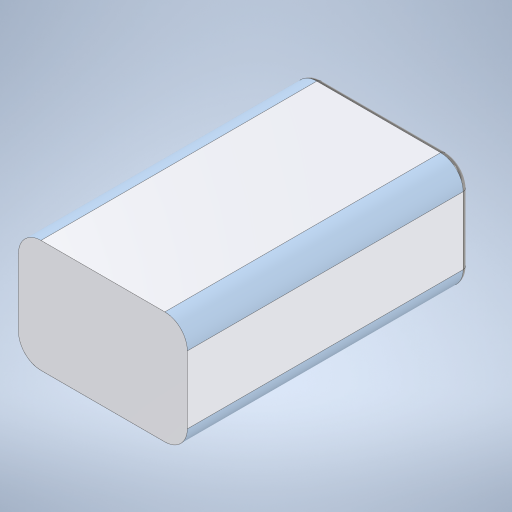
# Autodesk Inventor part: battery eg 26
Saved by Autodesk Inventor 2023 (Build 270158000, 158)
## iProperties
Created: 2023-10-16
Part Number: battery eg 26
Material: Generic
Document SubType Name: Modeling
Designer: user
Density: 1 g/cm^3
Appearance: Default
Author: user
Autodesk Inventor part; units mm, degrees
ref_plane "YZ Plane" through (0, 0, 0) normal (1, 0, 0) x (0, 1, 0)
ref_plane "XZ Plane" through (0, 0, 0) normal (0, 1, 0) x (-1, 0, 0)
ref_plane "XY Plane" through (0, 0, 0) normal (0, 0, 1) x (1, 0, 0)
sketch "Sketch1" plane through (0, 0, 0) normal (0, 0, 1) x (1, 0, 0)
  line L0 (0, 0) -> (150, 0)
  line L1 (150, 0) -> (150, 100)
  line L2 (150, 100) -> (0, 100)
  line L3 (0, 100) -> (0, 0)
  dimension "d0" = 150
  dimension "d1" = 100
  constraints: 8 end point, 2 parallel, 1 horizontal, 1 perpendicular
  measures "d0" distance of L1.end L2.end
  measures "d1" distance of L0.end L1.end
extrude "Extrusion1" add sketch "Sketch1" along normal blind 250
fillet "Fillet1" radius 20 1 edges at (150, 100, 125)
fillet "Fillet2" radius 20 1 edges at (150, 0, 125)
fillet "Fillet3" radius 20 1 edges at (0, 100, 125)
fillet "Fillet4" radius 20 1 edges at (0, 0, 125)
fillet "Fillet5" radius 5 8 edges at (5.8579, 94.1421, 0) (0, 50, 0) (5.8579, 5.8579, 0) (75, 0, 0) (144.1421, 5.8579, 0) (150, 50, 0) (144.1421, 94.1421, 0) (75, 100, 0)
sketch "Sketch2" plane through (20, 0, 250) normal (0, -1, 0) x (1, 0, 0)
  line L0 (110, 0) -> (110, -245) projected
  line L1 (0, -245) -> (0, 0) projected
  line L2 (110, -171.6757) -> (0, -171.6757)
  line L3 (0, -171.6757) -> (0, -166.6757)
  line L4 (0, -166.6757) -> (110, -166.6757)
  line L5 (110, -166.6757) -> (110, -171.6757)
  line L6 (95.3863, -226.2308) -> (70.3863, -226.2308)
  line L7 (70.3863, -226.2308) -> (70.3863, -221.2308)
  line L8 (70.3863, -221.2308) -> (95.3863, -221.2308)
  line L9 (95.3863, -221.2308) -> (95.3863, -226.2308)
  line L10 (37.9599, -226.2308) -> (12.9599, -226.2308)
  line L11 (12.9599, -226.2308) -> (12.9599, -221.2308)
  line L12 (12.9599, -221.2308) -> (37.9599, -221.2308)
  line L13 (37.9599, -221.2308) -> (37.9599, -226.2308)
  line L14 (27.9599, -236.2308) -> (22.9599, -236.2308)
  line L15 (22.9599, -236.2308) -> (22.9599, -211.2308)
  line L16 (22.9599, -211.2308) -> (27.9599, -211.2308)
  line L17 (27.9599, -211.2308) -> (27.9599, -236.2308)
  point P0 (-20, -250)
  point P1 (27.9599, -226.2308)
  point P2 (27.9599, -221.2308)
  point P3 (22.9599, -221.2308)
  point P4 (22.9599, -226.2308)
  dimension "d9" = 25
  dimension "d10" = 5
  dimension "d11" = 5
  dimension "d12" = 25
  dimension "d13" = 10
  dimension "d14" = 10
  dimension "d15" = 5
  dimension "d16" = 25
  dimension "d17" = 5
  constraints: 32 end point, 8 parallel, 4 horizontal, 4 perpendicular, 2 point on line, 1 coincident
  measures "d9" distance of L7.end L8.end
  measures "d10" distance of L6.end L7.end
  measures "d11" distance between parallel lines of L2 L4
  measures "d12" distance of L11.end L12.end
  measures "d13" horizontal distance of L14.start L10.start
  measures "d14" distance from line of L10 L14.start
  measures "d15" distance of L15.end L16.end
  measures "d16" distance of L14.end L15.end
  measures "d17" distance of L10.end L11.end
extrude "Extrusion2" add sketch "Sketch2" along normal blind 5
sketch "Sketch3" plane through (0, 0, 0) normal (0, 0, -1) x (-1, 0, 0)
  line L0 (-20, 100) -> (-130, 100) projected
  line L1 (-150, 80) -> (-150, 20) projected
  circle A0 centre (-110, 50) radius 12.5
  circle A1 centre (-40, 51.4507) radius 12.5
  point P0 (0, 0)
  point P1 (-150, 50)
  dimension "d20" = 50
  dimension "d21" = 40
  dimension "d22" = 70
  dimension "d23" = 25
  dimension "d24" = 25
  constraints: 2 centre point, 2 coincident, 1 midpoint
  measures "d20" distance from line of L0 point (-110, 50)
  measures "d21" distance of point (-150, 50) point (-110, 50)
  measures "d22" horizontal distance of point (-110, 50) point (-40, 51.451)
  measures "d23" diameter of A1
  measures "d24" diameter of A0
extrude "Extrusion3" add sketch "Sketch3" along normal blind 3
sketch "Sketch4" plane through (110, 50, -3) normal (0, 0, -1) x (-1, 0, 0)
  circle A0 centre (0, 0) radius 7.2404
  circle A1 centre (70, 1.4507) radius 12.5 projected
  circle A2 centre (70, 1.4507) radius 7.5
  point P0 (110, -50)
  dimension "d27" = 15
  constraints: 2 centre point, 1 coincident
  measures "d27" diameter of A2
extrude "Extrusion4" add sketch "Sketch4" along normal blind 15 contours A0 | A2
sketch "Sketch5" plane through (110, 50, -18) normal (0, 0, -1) x (-1, 0, 0)
  circle A0 centre (0, 0) radius 7.2404 projected
  circle A1 centre (0, 0) radius 10
  circle A2 centre (70, 1.4507) radius 7.5 projected
  circle A3 centre (70, 1.4507) radius 8.5
  point P0 (110, -50)
  dimension "d30" = 20
  dimension "d31" = 17
  constraints: 2 centre point, 2 coincident
  measures "d30" diameter of A1
  measures "d31" diameter of A3
extrude "Extrusion5" add sketch "Sketch5" along normal blind 4 contours A0 | A1 | A2 | A3
sketch "Sketch6" plane through (110, 50, -22) normal (0, 0, -1) x (-1, 0, 0)
  circle A0 centre (0, 0) radius 10 projected
  point P0 (110, -50)
  constraints: 1 coincident
hole "Hole1" at (110, 50, -22) direction (0, 0, 1) diameter 10.106 depth 28 tip angle 118 thread size "M12x1.75" class "6H" standard "ISO Metric profile"
sketch "Sketch7" plane through (40, 51.4507, -22) normal (0, 0, -1) x (-1, 0, 0)
  circle A0 centre (0, 0) radius 8.5 projected
  point P0 (40, -51.4507)
  constraints: 1 coincident
hole "Hole2" at (40, 51.4507, -22) direction (0, 0, 1) diameter 10.647 depth 28 tip angle 118 thread size "M12x1.25" class "6H" standard "ISO Metric profile"
sketch "Sketch8" plane through (0, 20, 250) normal (-1, 0, 0) x (0, 0, 1)
  line L0 (-245, 80) -> (-245, 60) projected
  line L1 (-245, 60) -> (-73.5714, 60) construction
  line L2 (-73.5714, 60) -> (-73.5714, 0) construction
  line L3 (-73.5714, 0) -> (-245, 0) construction
  line L4 (-245, 0) -> (-245, 60) construction
  line L5 (-245, 0) -> (-245, 60) projected
  point P0 (-250, -20)
  constraints: 1 collinear, 2 other
decal "Decal1"
sketch "Sketch9" plane through (20, 100, 250) normal (0, 1, 0) x (1, 0, 0)
  line L0 (0, 250) -> (110, 250) projected
  circle A0 centre (57.15, 250) radius 9.5
  point P0 (-20, 250)
  dimension "d50" = 19
  constraints: 1 centre point, 1 point on line
  measures "d50" diameter of A0
sketch "Sketch10" plane through (20, 0, 5) normal (0, -1, 0) x (1, 0, 0)
  line L0 (0, -5) -> (110, -5) projected
  circle A0 centre (57.15, -5) radius 9.5
  point P0 (-20, -5)
  point P1 (66.65, -5)
  point P2 (47.65, -5)
  dimension "d51" = 19
  constraints: 1 centre point, 1 point on line
  measures "d51" diameter of A0
extrude "Extrusion6" cut sketch "Sketch10" against normal blind 50 contours A0 L0 picked at (56.7683, -1.8564)
body "Solid1"
